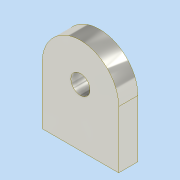
# Autodesk Inventor part: M1
Saved by Autodesk Inventor 2021 (Build 250183000, 183)
## iProperties
Created: 2022-01-10
Part Number: M1
Material: Generic
Document SubType Name: Modeling
Designer: student
Density: 1 g/cm^3
Appearance: Silver
Author: student
Autodesk Inventor part; units mm, degrees
ref_plane "YZ Plane" through (0, 0, 0) normal (1, 0, 0) x (0, 1, 0)
ref_plane "XZ Plane" through (0, 0, 0) normal (0, 1, 0) x (-1, 0, 0)
ref_plane "XY Plane" through (0, 0, 0) normal (0, 0, 1) x (1, 0, 0)
sketch "Sketch1" plane through (0, 0, 0) normal (0, 0, 1) x (1, 0, 0)
  line L0 (5.1301, 15) -> (5.1301, 0)
  line L1 (5.1301, 0) -> (-14.8699, 0)
  line L2 (-14.8699, 0) -> (-14.8699, 15)
  arc A0 (5.1301, 15) -> (-14.8699, 15) centre (-4.8699, 15) ccw
  circle A1 centre (-4.8699, 15) radius 2.5
  point P0 (0, 0)
  dimension "d0" = 15
  dimension "d1" = 20
  dimension "d2" = 10
  dimension "d5" = 5
  constraints: 6 end point, 2 centre point, 2 point on circle, 1 coincident, 1 parallel
  measures "d0" distance of L1.end L2.end
  measures "d1" distance of L0.end L1.end
  measures "d2" distance of L0.start A0.centre
  measures "d5" diameter of A1
extrude "Extrusion1" add sketch "Sketch1" along normal blind 5
body "Solid1"
